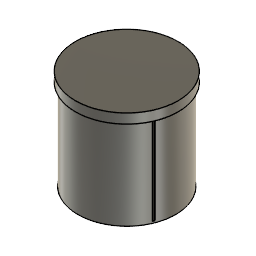
PillPod (Autodesk Fusion 360 design; units mm, degrees)
Autodesk Fusion 360 part; units mm, degrees
note: some values were not read from the file. Set by a fixed rule: which face or edge a step refers to.
sketch "Sketch1" plane through (0, 0, 0) normal (0, 0, 1) x (1, 0, 0)
  circle A0 centre (0, 0) radius 25.4
  circle A1 centre (0, 0) radius 2.55
  ellipse E0 centre (0, -16) end of major axis (0, -22) minor radius 13
  line L0 (0, -10) -> (0, -22) construction
  line L1 (-13, -16) -> (13, -16) construction
  circle A2 centre (0, 0) radius 24.13
  dimension "d1" = 50.8
  dimension "d2" = 5.1
  dimension "d5" = 48.26
  constraint coincident A0.centre A1.centre
  constraint concentric A0 A1
  constraint coincident E0 L0.start
  constraint coincident E0 L0.end
  constraint coincident E0 L1.start
  constraint coincident E0 L1.end
  constraint vertical L0
  measures "d1" diameter of A0
  measures "d2" diameter of A1
  measures "d5" diameter of A2
extrude "Extrude1" add sketch "Sketch1" along normal blind 1 contours A0 | A2 makes body 1
extrude "Extrude2" add sketch "Sketch1" along normal blind 50.8 contours A0 bodies 1
ref_plane "WorkPlane1" through (0, 25.4, 12.6225) normal (0, 1, 0) x (1, 0, 0)
sketch "Sketch3" plane through (0, 25.4, 0) normal (0, 1, 0) x (1, 0, 0)
  line L0 (-25.4, 0) -> (25.4, 0)
  line L1 (3, 0) -> (-3, 0)
  line L2 (3, 0) -> (3, -10.16)
  line L3 (3, -10.16) -> (-3, -10.16)
  line L4 (-3, -10.16) -> (-3, 0)
  line L5 (-3, 0) -> (3, 0)
  line L6 (3, 0) -> (3, -10.16)
  dimension "d9" = 6
  dimension "d10" = 10.16
  constraint midpoint L1 origin
  constraint parallel L0 L1
  constraint perpendicular L1 L2
  constraint horizontal L3
  constraint vertical L4
  constraint horizontal L5
  constraint vertical L6
  measures "d9" distance of L1.start L1.end
  measures "d10" distance of L1.start L2.end
extrude "Extrude3" add sketch "Sketch3" along normal blind 2.54 separate body makes body 2
extrude "Extrude4" add 1 faces at (-1, 25.4, 3.3867) along direction (0, -1, 0) blind 0.2 on bodies 2 bodies 1 2
sketch "Sketch4" plane through (0, 0, 0) normal (0, 0, 1) x (1, 0, 0)
  circle A0 centre (0, 0) radius 2.55
  point P0 (-2.55, 0)
  constraint coincident A0.centre origin
  constraint coincident A0 P0
extrude "Extrude5" add sketch "Sketch4" along normal blind 10 separate body makes body 3
move_body "Move1" bodies 3 to x (1, 0, 0) y (0, 1, 0) z (0, 0, 1) at (65.2873, -3.5214, 0)
move_face "OffsetFaces1" offset 1 1 faces at (65.978, -1.0667, 6.6667) on bodies 3
ref_plane "WorkPlane2" through (65.2873, -3.5214, 0) normal (0, 0, -1) x (-1, 0, 0)
sketch "Sketch5" plane through (0, 0, 0) normal (0, 0, -1) x (-1, 0, 0)
  circle A0 centre (-65.2873, -3.5214) radius 3.55
  circle A1 centre (-65.2873, -3.5214) radius 2.5
  line L0 (-66.7873, -1.5214) -> (-66.7873, -5.5214)
  line L1 (-63.7873, -1.5214) -> (-63.7873, -5.5214)
  circle A2 centre (-65.2873, -3.5214) radius 24.13
  line L2 (-65.2873, 18.0686) -> (-65.2873, -25.1114)
  line L3 (-66.0373, -25.1114) -> (-64.5373, -25.1114)
  line L4 (-66.0373, -3.5214) -> (-64.5373, -3.5214)
  line L5 (-64.5373, -3.5214) -> (-66.0373, -3.5214)
  line L6 (-66.0373, -3.5214) -> (-66.0373, -25.1114)
  line L7 (-66.0373, -25.1114) -> (-64.5373, -25.1114)
  line L8 (-64.5373, -25.1114) -> (-64.5373, -3.5214)
  point P0 (-65.2873, -3.5214)
  point P1 (-65.2873, -3.5214)
  point P2 (-65.2873, -3.5214)
  dimension "d19" = 5
  dimension "d23" = 48.26
  dimension "d24" = 43.18
  dimension "d25" = 1.5
  dimension "d26" = 1.5
  constraint concentric A0 A1
  constraint coincident P2 P0
  constraint coincident A1 L0.end
  constraint coincident A1 L1.end
  constraint concentric A1 A2
  constraint midpoint L2 P2
  constraint parallel L0 L2
  constraint midpoint L2.end L3
  constraint perpendicular L2 L3
  constraint midpoint L4 P2
  constraint coincident P2 P1
  constraint perpendicular L2 L4
  constraint horizontal L5
  constraint vertical L6
  constraint horizontal L7
  constraint vertical L8
  measures "d19" diameter of A1
  measures "d23" diameter of A2
  measures "d24" distance of L2.start L2.end
  measures "d25" distance of L3.start L3.end
  measures "d26" distance of L4.start L4.end
extrude "Extrude6" cut sketch "Sketch5" against normal blind 6.1 contours A1 L0 L2 L4 L5 L6 | A1 L1 L2 L4 L5 L8 | A1 L2 L4 L5 L8 | A1 L2 L4 L5 L6 bodies 3
extrude "Extrude8" add 1 faces at (66.1766, -4.0349, 10) along direction (0, 0, 1) blind 3 on bodies 3 bodies 3
extrude "Extrude9" add sketch "Sketch5" against normal blind 13 separate body contours A0 L2 L3 L7 L8 | A0 L2 L3 L6 L7 makes body 4
pattern_circular "C-Pattern1" count 6 over 360 about axis through (65.2873, -3.5214, -6.5) along (0, 0, 1) of bodies 4 makes body 5 at (78.379, -11.9459, 8.6667) makes body 6 at (79.129, 3.604, 8.6667) makes body 7 at (66.0373, 12.0285, 8.6667) makes body 8 at (52.1957, 4.9031, 8.6667) makes body 9 at (51.4457, -10.6469, 8.6667)
combine "Combine1" operation add target body 8 tool bodies 6 3 7 4 5 9
ref_plane "WorkPlane3" through (65.2873, -3.5214, 13) normal (0, 0, 1) x (-0.5, -0.866025, 0)
sketch "Sketch6" plane through (0, 0, 13) normal (0, 0, 1) x (1, 0, 0)
  circle A0 centre (65.2873, -3.5214) radius 3.55
extrude "Extrude10" add sketch "Sketch6" along normal blind 3 bodies 8
ref_plane "WorkPlane4" through (65.2873, -3.5214, 16) normal (0, 0, 1) x (1, 0, 0)
sketch "Sketch7" plane through (0, 0, 16) normal (0, 0, 1) x (1, 0, 0)
  circle A0 centre (65.2873, -3.5214) radius 3.55
  circle A1 centre (65.2873, -3.5214) radius 2.5
  dimension "d39" = 5
  constraint concentric A0 A1
  measures "d39" diameter of A1
extrude "Extrude11" add sketch "Sketch7" along normal blind 1 contours A1 bodies 8
extrude "Extrude12" add 1 faces at (64.672, -3.5051, 17) along direction (0, 0, 1) blind 6 on bodies 8 bodies 8
ref_plane "WorkPlane5" through (65.2873, -3.5214, 23) normal (0, 0, 1) x (1, 0, 0)
sketch "Sketch8" plane through (0, 0, 23) normal (0, 0, 1) x (1, 0, 0)
  circle A0 centre (65.2873, -3.5214) radius 2.5
  arc A1 (63.7873, -5.5214) -> (66.7873, -5.5214) centre (65.2873, -3.5214) ccw
  line L0 (65.2873, -1.0214) -> (65.2873, -6.0214)
  point P0 (65.2873, -3.5214)
  constraint midpoint L0 P0
  constraint coincident P0 A0.centre
  constraint coincident A1 L0.end
  constraint vertical L0
extrude "Extrude13" cut sketch "Sketch8" against normal blind 3 contours A0 A1 L0 picked at (63.8731, -2.8161) bodies 8
ref_plane "WorkPlane6" through (0, 0, 17) normal (0, 0, 1) x (1, 0, 0)
sketch "Sketch9" plane through (0, 0, 17) normal (0, 0, 1) x (1, 0, 0)
  circle A0 centre (0, 0) radius 24.13
  circle A1 centre (0, 0) radius 2.55
  ellipse E0 centre (0, -16) end of major axis (13, -16) minor radius 6
  circle A2 centre (0, 0) radius 24.13
  circle A3 centre (0, 0) radius 23.876
  dimension "d48" = 48.26
  dimension "d49" = -0.254
  constraint concentric A0 A2
  measures "d48" diameter of A2
extrude "Extrude14" add sketch "Sketch9" against normal blind 16 contours A0 A2 bodies 1
move_face "OffsetFaces2" offset 1 1 faces at (-23.7574, 2.3773, 6.3333) on bodies 1
sketch "Sketch10" plane through (0, 0, 0) normal (0, 0, 1) x (1, 0, 0)
  circle A0 centre (0, 0) radius 24
  circle A1 centre (0, 0) radius 2.55
  ellipse E0 centre (0, -16) end of major axis (13, -16) minor radius 6
  dimension "d53" = 48
  constraint coincident A0.centre A1.centre
  measures "d53" diameter of A0
move_body "Move2" bodies 1 to x (1, 0, 0) y (0, 1, 0) z (0, 0, 1) at (41.9523, 37.3422, 0)
sketch "Sketch11" plane through (0, 0, 0) normal (0, 0, 1) x (1, 0, 0)
  circle A0 centre (0, 0) radius 3.55
  dimension "d57" = 7.1
  constraint coincident A0.centre origin
  measures "d57" diameter of A0
move_body "Move4" bodies 8 to x (1, 0, 0) y (0, 1, 0) z (0, 0, 1) at (-23.3798, 40.8724, 0)
move_body "Move5" bodies 8 to x (1, 0, 0) y (0, 1, 0) z (0, 0, 1) at (0, 0, 1)
ref_plane "WorkPlane8" through (41.9523, 37.3422, 50.8) normal (0, 0, 1) x (1, 0, 0)
sketch "Sketch13" plane through (0, 0, 50.8) normal (0, 0, 1) x (1, 0, 0)
  circle A0 centre (41.9523, 37.3422) radius 25.4
  circle A1 centre (41.9523, 37.3422) radius 26.65
  circle A2 centre (41.9523, 37.3422) radius 25.65
  dimension "d74" = 1.25
  dimension "d77" = 0.25
extrude "Extrude21" add sketch "Sketch13" along normal blind 5 separate body contours A1 makes body 10
ref_plane "WorkPlane9" through (41.9523, 37.3422, 55.8) normal (0, 0, 1) x (1, 0, 0)
sketch "Sketch14" plane through (0, 0, 55.8) normal (0, 0, 1) x (1, 0, 0)
  circle A0 centre (41.9523, 37.3422) radius 25.65
extrude "Extrude22" add sketch "Sketch14" against normal blind 1 bodies 10
move_body "Move9" bodies 10 to x (1, 0, 0) y (0, 1, 0) z (0, 0, 1) at (0, 0, -4)
move_face "OffsetFaces4" offset -0.2 5 faces at (40.4075, 38.0177, 3.0333) (43.0013, 39.599, 5.0667) (43.4075, 38.0177, 3.0333) (42.893, 35.0534, 5.0667) (44.4991, 37.215, 0.6667) on bodies 1 8
extrude "Extrude23" cut 1 faces at (60.7945, 23.0448, 17) along direction (0, 0, -1) blind 16 on bodies 1 bodies 1
move_body "Move10" bodies 8 to x (1, 0, 0) y (0, 1, 0) z (0, 0, 1) at (-60, 0, 0)
extrude "Extrude24" cut 1 faces at (-17.3344, 37.6972, 24) along direction (0, 0, -1) blind 3 on bodies 8 bodies 8
extrude "Extrude25" cut 1 faces at (-17.7148, 37.8894, 21) along direction (0, 0, -1) blind 4 on bodies 8 bodies 8
extrude "Extrude26" cut 6 faces at (-31.5377, 45.2105, 14) (-18.1764, 52.9247, 14) (-4.6472, 45.2105, 14) (-4.6472, 29.4915, 14) (-18.0086, 21.7773, 14) (-31.6216, 29.6368, 14) along direction (0, 0, -1) blind 17 on bodies 8 bodies 8
extrude "Extrude27" cut 1 faces at (-18.5248, 38.4525, 17) along direction (0, 0, -1) blind 8 on bodies 8 bodies 8
ref_plane "WorkPlane10" through (-18.0925, 37.351, 1) normal (0, 0, -1) x (0.5, 0.866025, 0)
sketch "Sketch15" plane through (0, 0, 1) normal (0, 0, -1) x (-1, 0, 0)
  circle A0 centre (18.0925, 37.351) radius 3.55
  circle A1 centre (18.0925, 37.351) radius 23.495
  dimension "d95" = 46.99
  constraint concentric A0 A1
  measures "d95" diameter of A1
extrude "Extrude28" add sketch "Sketch15" against normal blind 8 bodies 8
chamfer "Chamfer1" distance 23 angle 15 1 edges at (3.8126, 45.8471, 9) measured on face at (-10.3483, 36.1837, 9) on bodies 8
sketch "Sketch17" plane through (0, 0, 1) normal (0, 0, -1) x (1, 0, 0)
  circle A0 centre (-18.0925, -37.351) radius 23.495
  arc A1 (-16.3925, -35.2534) -> (-19.7925, -35.2534) centre (-18.0925, -37.351) ccw
  line L0 (-16.3925, -35.2534) -> (-16.3925, -39.4486)
  arc A2 (-19.7925, -39.4486) -> (-16.3925, -39.4486) centre (-18.0925, -37.351) ccw
  line L1 (-19.7925, -39.4486) -> (-19.7925, -35.2534)
  line L2 (5.4025, -33.351) -> (5.4025, -41.351)
  line L3 (5.4025, -33.351) -> (-2.5975, -33.351)
  line L4 (-2.5975, -33.351) -> (5.4025, -33.351)
  line L5 (5.4025, -33.351) -> (5.4025, -41.351)
  line L6 (5.4025, -41.351) -> (-2.5975, -41.351)
  line L7 (-2.5975, -41.351) -> (-2.5975, -33.351)
  point P0 (5.4025, -37.351)
  point P1 (5.4025, -37.351)
  dimension "d100" = 8
  dimension "d101" = 8
  constraint midpoint L2 P1
  constraint coincident P1 P0
  constraint vertical L2
  constraint perpendicular L2 L3
  constraint horizontal L4
  constraint vertical L5
  constraint horizontal L6
  constraint vertical L7
  measures "d100" distance of L2.start L2.end
  measures "d101" distance of L2.start L3.end
extrude "Extrude29" cut sketch "Sketch17" against normal blind 15 contours A0 L3 L4 L6 L7 picked at (0.0692, -37.351) bodies 8
sketch "Sketch18" plane through (0, 0, 1) normal (0, 0, 1) x (-1, 0, 0)
  circle A0 centre (-41.9523, -37.3422) radius 24.13
  circle A1 centre (-41.9523, -37.3422) radius 2.75
  ellipse E0 centre (-41.9523, -21.3422) end of major axis (-54.9523, -21.3422) minor radius 6
  line L0 (-41.9523, -21.3422) -> (-41.9523, -27.3438)
  line L1 (-19.9912, -27.3438) -> (-63.9134, -27.3438)
  line L2 (-41.9523, -27.3438) -> (-19.9912, -27.3438) construction
  line L3 (-63.9134, -27.3438) -> (-64.4134, -27.3438)
  line L4 (-19.9912, -27.3438) -> (-19.4912, -27.3438)
  line L5 (-19.4912, -27.3438) -> (-64.4134, -27.3438)
  line L6 (-64.4134, -27.3438) -> (-64.4134, -28.3438)
  line L7 (-64.4134, -28.3438) -> (-19.4912, -28.3438)
  line L8 (-19.4912, -28.3438) -> (-19.4912, -27.3438)
  dimension "d104" = 180
  dimension "d105" = 0.5
  dimension "d106" = 0.5
  dimension "d107" = 1
  constraint vertical L0
  constraint coincident E0.centre L0.start
  constraint midpoint L0.end L1
  constraint horizontal L2
  constraint coincident A0 L1.end
  constraint parallel L1 L3
  constraint parallel L1 L4
  constraint horizontal L5
  constraint vertical L6
  constraint horizontal L7
  constraint vertical L8
  measures "d104" angle of L1 L2
  measures "d105" distance of L1.end L3.end
  measures "d106" distance of L1.start L4.end
  measures "d107" distance of L4.end L7.end
extrude "Extrude30" cut sketch "Sketch18" along normal blind 80 contours A0 L4 L5 L7 L8 | A0 L1 L5 L7 | A0 L3 L5 L6 L7 bodies 1
extrude "Extrude31" add sketch "Sketch18" along normal blind 50 separate body contours A0 L4 L5 L7 L8 | A0 L1 L5 L7 | A0 L3 L5 L6 L7 makes body 11
move_body "Move11" bodies 11 to x (1, 0, 0) y (0, 1, 0) z (0, 0, 1) at (-60, 0, 0)
sketch "Sketch19" plane through (0, 27.3438, 0) normal (0, -1, 0) x (1, 0, 0)
  line L0 (-40.5088, 1) -> (4.4134, 1)
  line L1 (4.4134, 1) -> (4.4134, 51)
  line L2 (4.4134, 51) -> (-40.5088, 51)
  line L3 (-40.5088, 51) -> (-40.5088, 1)
  line L4 (3.2, 1) -> (3.2, 3)
  line L5 (-39.4, 1) -> (-39.4, 3)
  arc A0 (3.2, 3) -> (-39.4, 3) centre (-18.1, -49.9225) ccw
  point P0 (-16.3925, 7.1)
  constraint coincident L0 L4.start
  constraint perpendicular L0 L4
  constraint coincident L0 L5.start
  constraint perpendicular L0 L5
  constraint coincident A0 P0
extrude "Extrude32" cut sketch "Sketch19" against normal blind 3 contours L0 L4 L5 A0 bodies 11
extrude "Extrude33" cut 1 faces at (-18.0651, 28.3438, 36.3752) along direction (0, -1, 0) blind 0.05 on bodies 11 bodies 11
extrude "Extrude34" cut 1 faces at (4.4134, 27.6604, 17.6667) along direction (-1, 0, 0) blind 0.025 on bodies 11 bodies 11
extrude "Extrude35" cut 1 faces at (-40.5088, 27.9771, 17.6667) along direction (1, 0, 0) blind 0.025 on bodies 11 bodies 11
move_body "Move12" bodies 8 11 to x (1, 0, 0) y (0, 1, 0) z (0, 0, 1) at (60, 0, 0)
move_face "OffsetFaces5" offset -0.25 3 faces at (61.7743, 33.351, 1.8056) (57.4025, 37.351, 2.3269) (61.7743, 41.351, 1.8056) on bodies 8
move_face "OffsetFaces6" offset -2 1 faces at (32.245, 27.6604, 6.3026) on bodies 11
move_face "OffsetFaces7" offset 10 2 faces at (64.3884, 27.6604, 17.6667) (19.5162, 27.6604, 17.6667) on bodies 11
extrude "Extrude36" cut 1 faces at (31.1403, 27.6604, 51) along direction (0, 0, -1) blind 1 on bodies 11 bodies 11
extrude "Extrude37" cut 1 faces at (31.1403, 27.6604, 50) along direction (0, 0, -1) blind 4 on bodies 11 bodies 11
extrude "Extrude38" cut 1 faces at (9.5162, 27.6604, 31) along direction (1, 0, 0) blind 11 on bodies 11 bodies 1 8 11
extrude "Extrude39" cut 1 faces at (74.3884, 27.9771, 31) along direction (-1, 0, 0) blind 11 on bodies 11 bodies 1 8 11
move_face "OffsetFaces8" offset 11 2 faces at (20.5162, 27.6604, 31) (63.3884, 27.9771, 31) on bodies 11
extrude "Extrude40" cut 1 faces at (31.1403, 27.6604, 46) along direction (0, 0, 1) blind 6 on bodies 11 bodies 1
extrude "Extrude41" cut 1 faces at (74.3884, 27.9771, 31) along direction (-1, 0, 0) blind 2 on bodies 11 bodies 11
extrude "Extrude42" cut 1 faces at (9.5162, 27.6604, 31) along direction (1, 0, 0) blind 2 on bodies 11 bodies 11
move_face "OffsetFaces9" offset -0.5 2 faces at (20.6, 27.6604, 2.3833) (63.2, 27.9771, 3.7667) on bodies 11
extrude "Extrude43" cut 1 faces at (72.3884, 27.9771, 31) along direction (-1, 0, 0) blind 7 on bodies 11 bodies 11
extrude "Extrude44" cut 1 faces at (11.5162, 27.6604, 31) along direction (1, 0, 0) blind 7 on bodies 11 bodies 11
extrude "Extrude45" add 1 faces at (34.1403, 27.6604, 46) along direction (0, 0, 1) blind 4 on bodies 11 bodies 11
named bodies: "Pod", "Agitator", "Fins", "Fins (1)", "Fins (2)", "Fins (3)", "Fins (5)", "Lid", "Seperator"
